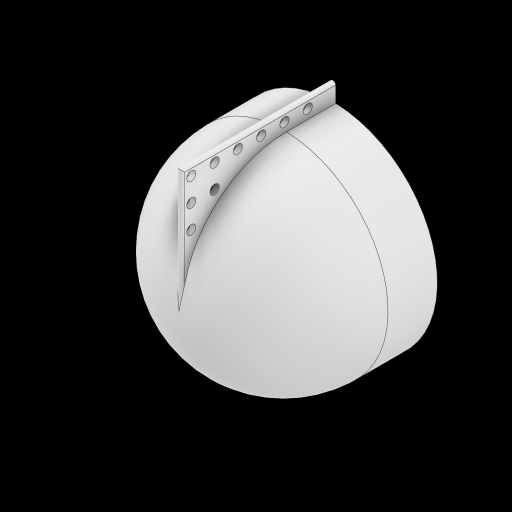
# Autodesk Inventor part: FrontCapV1
Saved by Autodesk Inventor 2024 (Build 280153000, 153)
## iProperties
Created: 2026-04-10
Part Number: FrontCapV1
Material: PVC-Piping
Document SubType Name: Modeling
Designer: Tanner
Density: 1.4 g/cm^3
Appearance: Smooth - White
Author: Tanner
## iProperties of the stored document FrontCapV1_3DPrint.ipt
Created: 2026-04-13
Part Number: FrontCapV1_3DPrint
Material: Generic
Document SubType Name: Modeling
Designer: Tanner
Density: 1 g/cm^3
Appearance: Default
Author: Tanner
Autodesk Inventor part; units mm, degrees
ref_plane "YZ Plane" through (0, 0, 0) normal (1, 0, 0) x (0, 1, 0)
ref_plane "XZ Plane" through (0, 0, 0) normal (0, 1, 0) x (-1, 0, 0)
sketch "Sketch1" plane through (0, 0, 0) normal (1, 0, 0) x (0, 1, 0)
  line L0 (107.6, 0) -> (-107.6, 0) construction
  line L1 (108.1, 0) -> (108.1, -40)
  line L2 (108.1, -40) -> (112.1, -40)
  line L3 (112.1, -40) -> (112.1, 12.9)
  line L4 (0, 0) -> (0, 125)
  arc A0 (112.1, 12.9) -> (0, 125) centre (0, 12.9) ccw
  line L5 (108.1, 0) -> (0, 0)
  line L6 (98.1, 0) -> (98.1, 12.9)
  arc A1 (98.1, 12.9) -> (0, 111) centre (0, 12.9) ccw
  line L7 (99.6, 0) -> (99.6, -254) construction
  line L8 (107.6, -254) -> (107.6, 0) construction
  dimension "d0" = 125
  dimension "d2" = 40
  dimension "d5" = 10
  dimension "d8" = 0.5
  dimension "d9" = 4
  constraints: 16 end point, 4 point on circle, 4 vertical, 3 perpendicular, 2 centre point, 2 point on line, 1 collinear, 1 concentric, 1 horizontal alignment, 1 line through centre, 1 tangent, 4 other
  measures "d0" distance of L4.start L4.end
  measures "d2" distance between parallel lines of L5 L2
  measures "d5" distance between parallel lines of L1 L6
  measures "d8" distance between parallel lines of L8 L1
  measures "d9" distance between parallel lines of L1 L3
revolve "Revolution1" add sketch "Sketch1" angle 360 about axis through (0, 0, 0) along (0, 0, 1) contours L5 L6 A1 L4 A0 L3 L2 L1
ref_plane "Work Plane1" through (0, 108.1, -624) normal (0, 0, 1) x (1, 0, 0)
sketch "Sketch6" plane through (0, 0, 0) normal (1, 0, 0) x (0, 1, 0)
  arc A0 (112.1, 12.9) -> (-112.1, 12.9) centre (0, 12.9) ccw construction
  arc A1 (98.1, 12.9) -> (-98.1, 12.9) centre (0, 12.9) ccw construction
  line L0 (98.1, 12.9) -> (98.1, 0) construction
  line L1 (112.1, -40) -> (112.1, 12.9) construction
  line L2 (108.1, 0) -> (108.1, -40) construction
  line L3 (108.1, 0) -> (-108.1, 0) construction
  line L4 (112.1, 12.9) -> (-112.1, 12.9) construction
  arc A2 (108.1, 12.9) -> (0, 121) centre (0, 12.9) ccw
  line L5 (0, 125) -> (132.1, 125)
  line L6 (132.1, 125) -> (132.1, -40)
  line L7 (132.1, -40) -> (108.1, -40)
  line L8 (108.1, 12.9) -> (108.1, -40)
  line L9 (112.1, -40) -> (-112.1, -40) projected
  line L10 (0, 125) -> (0, 121)
  point P0 (0, 0)
  point P1 (0, 0)
  dimension "d33" = 20
  constraints: 10 end point, 3 perpendicular, 2 point on circle, 2 vertical alignment, 1 centre point, 1 concentric, 1 horizontal, 1 midpoint, 1 point on line, 1 tangent, 1 vertical
  measures "d33" distance between parallel lines of L6 L1
extrude "Extrusion5" add sketch "Sketch6" along normal mid plane 6
sketch "Sketch7" plane through (3, 0, 0) normal (1, 0, 0) x (0, 0, -1)
  arc A0 (-12.9, 112.0599) -> (-124.9599, 0) centre (-12.9, 0) ccw construction
  line L0 (40, 112.0599) -> (-12.9, 112.0599) construction
  line L1 (40, 112.0599) -> (40, 132.1) construction
  line L2 (40, 132.1) -> (-125, 132.1) construction
  line L3 (-125, 132.1) -> (-125, 0) construction
  circle A1 centre (-115, 72.1) radius 5
  circle A2 centre (-115, 97.1) radius 5
  circle A3 centre (-115, 122.1) radius 5
  circle A4 centre (-90, 122.1) radius 5
  circle A5 centre (-65, 122.1) radius 5
  circle A6 centre (-40, 122.1) radius 5
  circle A7 centre (-15, 122.1) radius 5
  circle A8 centre (10, 122.1) radius 5
  circle A9 centre (-90, 97.1) radius 5
  line L4 (-125, 0) -> (-124.9599, 0) projected
  point P0 (0, 0)
  dimension "d37" = 10
  dimension "d38" = 10
  dimension "d39" = 10
  dimension "d40" = 10
  dimension "d41" = 10
  dimension "d42" = 10
  dimension "d43" = 10
  dimension "d44" = 10
  dimension "d45" = 10
  dimension "d46" = 25
  dimension "d47" = 25
  dimension "d50" = 25
  dimension "d51" = 25
  dimension "d52" = 25
  dimension "d53" = 25
  dimension "d54" = 10
  dimension "d55" = 25
  dimension "d56" = 10
  constraints: 9 centre point, 6 horizontal alignment, 3 vertical alignment
  measures "d37" diameter of A1
  measures "d38" diameter of A2
  measures "d39" diameter of A3
  measures "d40" diameter of A4
  measures "d41" diameter of A5
  measures "d42" diameter of A6
  measures "d43" diameter of A7
  measures "d44" distance from line of L2 A3.centre
  measures "d45" distance from line of L3 A3.centre
  measures "d46" distance of A3.centre A2.centre
  measures "d47" distance of A2.centre A1.centre
  measures "d50" distance of A3.centre A4.centre
  measures "d51" distance of A4.centre A5.centre
  measures "d52" distance of A5.centre A6.centre
  measures "d53" distance of A7.centre A6.centre
  measures "d54" diameter of A8
  measures "d55" distance of A7.centre A8.centre
  measures "d56" diameter of A9
extrude "Extrusion6" cut sketch "Sketch7" against normal through all
fillet "Fillet3" radius 3 4 edges at (3, 66.05, 125) (-3, 66.05, 125) (-3, 132.1, 42.5) (3, 132.1, 42.5)
body "Solid1"
